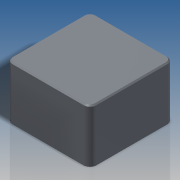
# Autodesk Inventor part: 99146-LtBluishGray
Saved by Autodesk Inventor 2016 SP2 (Build 200236200, 236)
## iProperties
Created: 2015-08-19
Part Number: 99146-LtBluishGray
Material: ABS Plastic
Document SubType Name: Modeling
Designer: D. Kohfeld
Mass: 0.365077 g
Surface Area: 2.94684 cm^2
Volume: 0.344412 cm^3
Density: 1.06 g/cm^3
Appearance: LtBluishGray
Author: D. Kohfeld
Autodesk Inventor part; units mm, degrees
ref_plane "YZ Plane" through (0, 0, 0) normal (1, 0, 0) x (0, 1, 0)
ref_plane "XZ Plane" through (0, 0, 0) normal (0, 1, 0) x (-1, 0, 0)
ref_plane "XY Plane" through (0, 0, 0) normal (0, 0, 1) x (1, 0, 0)
sketch "Sketch2" plane through (0, 0, 0) normal (0, 1, 0) x (-1, 0, 0)
  line L0 (-4.08, 4.08) -> (4.08, 4.08)
  line L1 (4.08, 4.08) -> (4.08, -4.08)
  line L2 (4.08, -4.08) -> (-4.08, -4.08)
  line L3 (-4.08, -4.08) -> (-4.08, 4.08)
  point P0 (0, 0)
  point P1 (0, 4.08)
  point P2 (-4.08, 0)
  dimension "d0" = 8.16
  constraints: 8 end point, 2 midpoint, 2 parallel, 2 perpendicular, 1 horizontal, 1 horizontal alignment, 1 vertical alignment
  measures "d0" distance between parallel lines of L2 L0
extrude "Extrusion1" add sketch "Sketch2" along normal mid plane 5.2
fillet "Fillet1" radius 0.6 4 edges at (-4.08, 0, 4.08) (4.08, 0, 4.08) (4.08, 0, -4.08) (-4.08, 0, -4.08)
chamfer "Chamfer1" distance 0.12 angle 45 8 edges at (0, 2.6, 4.08) (3.9043, 2.6, 3.9043) (4.08, 2.6, 0) (3.9043, 2.6, -3.9043) (0, 2.6, -4.08) (-3.9043, 2.6, -3.9043) (-4.08, 2.6, 0) (-3.9043, 2.6, 3.9043)
body "Solid1"
